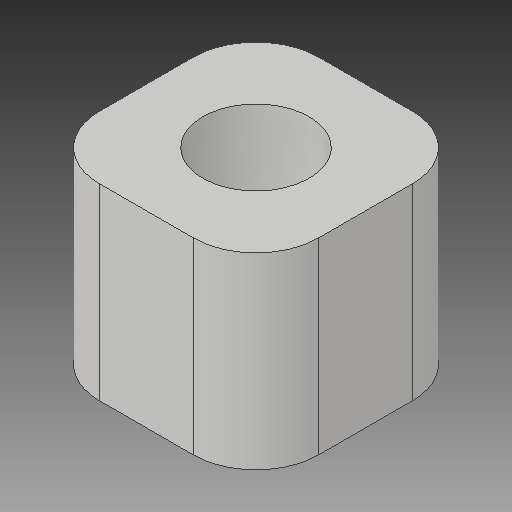
# Autodesk Inventor part: lcd_spacer
Saved by Autodesk Inventor 2019 (Build 230136000, 136)
## iProperties
Created: 2018-09-19
Part Number: lcd_spacer
Material: Generic
Document SubType Name: Modeling
Designer: Ax
Density: 1 g/cm^3
Appearance: Default
Mass: 0.218923 g
Surface Area: 2.84461 cm^2
Volume: 0.218923 cm^3
Author: Ax
Autodesk Inventor part; units mm, degrees
ref_plane "YZ Plane" through (0, 0, 0) normal (1, 0, 0) x (0, 1, 0)
ref_plane "XZ Plane" through (0, 0, 0) normal (0, 1, 0) x (-1, 0, 0)
ref_plane "XY Plane" through (0, 0, 0) normal (0, 0, 1) x (1, 0, 0)
sketch "Sketch1" plane through (0, 0, 0) normal (0, 1, 0) x (-1, 0, 0)
  circle A0 centre (0, 0) radius 1.7
  line L0 (-3.5, 3.5) -> (3.5, 3.5)
  line L1 (3.5, 3.5) -> (3.5, -3.5)
  line L2 (3.5, -3.5) -> (-3.5, -3.5)
  line L3 (-3.5, -3.5) -> (-3.5, 3.5)
  line L4 (-3.5, 3.5) -> (3.5, -3.5) construction
  line L5 (3.5, 3.5) -> (-3.5, -3.5) construction
  dimension "d0" = 3.4
  dimension "d1" = 7
  constraints: 12 end point, 2 midpoint, 2 parallel, 2 perpendicular, 1 centre point, 1 coincident, 1 horizontal
  measures "d0" diameter of A0
  measures "d1" distance of L0.end L1.end
extrude "Extrusion1" add sketch "Sketch1" along normal blind 6
fillet "Fillet1" radius 2 4 edges at (3.5, 3, 3.5) (3.5, 3, -3.5) (-3.5, 3, -3.5) (-3.5, 3, 3.5)
body "Solid1"
